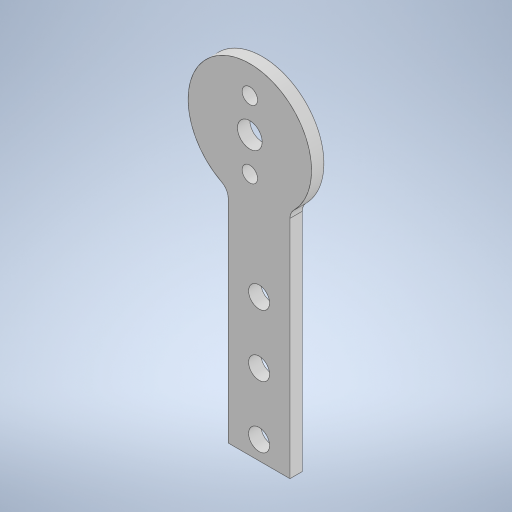
# Autodesk Inventor part: cutter_board_claws_endeffector_8_5_rotary-blade
Saved by Autodesk Inventor 2024 (Build 280153000, 153)
## iProperties
Created: 2025-06-01
Part Number: cutter_board_claws_endeffector_8_5_rotary-blade
Material: 一般
Document SubType Name: Modeling
Designer: 1412z
Density: 1 g/cm^3
Appearance: 既定
Author: 1412z
Autodesk Inventor part; units mm, degrees
ref_plane "YZ Plane" through (0, 0, 0) normal (1, 0, 0) x (0, 1, 0)
ref_plane "XZ Plane" through (0, 0, 0) normal (0, 1, 0) x (-1, 0, 0)
ref_plane "XY Plane" through (0, 0, 0) normal (0, 0, 1) x (1, 0, 0)
sketch "スケッチ1" plane through (0, 0, 0) normal (0, 0, 1) x (1, 0, 0)
  circle A0 centre (0, 0) radius 10
  line L0 (0, 0) -> (6.5, 0)
  line L1 (6.5, 0) -> (6.5, -45)
  line L2 (6.5, -45) -> (-3.5, -45)
  line L3 (-3.5, -45) -> (-3.5, 0)
  circle A1 centre (1.5, -22) radius 1.7
  circle A2 centre (1.5, -32) radius 1.7
  circle A3 centre (1.5, -42) radius 1.7
  circle A4 centre (0, 0) radius 5.5
  circle A5 centre (0, 5.5) radius 1.25
  circle A6 centre (0, -5.5) radius 1.25
  circle A7 centre (0, 0) radius 2
  point P0 (6.5, -7.5993)
  point P1 (-3.5, -9.3675)
  dimension "d0" = 20
  dimension "d3" = 6.5
  dimension "d4" = 45
  dimension "d5" = 10
  dimension "d6" = 3.4
  dimension "d7" = 3.4
  dimension "d8" = 3.4
  dimension "d9" = 11
  dimension "d10" = 2.5
  dimension "d11" = 2.5
  dimension "d12" = 4
  constraints: 8 centre point, 8 end point, 3 coincident, 3 perpendicular, 2 point on circle, 1 horizontal, 1 point on line
  measures "d0" diameter of A0
  measures "d3" distance of L0.start L0.end
  measures "d4" distance of L0.end L1.end
  measures "d5" distance of L1.end L2.end
  measures "d6" diameter of A1
  measures "d7" diameter of A2
  measures "d8" diameter of A3
  measures "d9" diameter of A4
  measures "d10" diameter of A5
  measures "d11" diameter of A6
  measures "d12" diameter of A7
extrude "押し出し1" add sketch "スケッチ1" along normal blind 2 contours A0 L1 L0 A4 A5 L3 | L3 A4 A6 L0 L1 A0 | A0 L1 L2 L3 | A4 A5 A6
fillet "フィレット1" radius 2 2 edges at (6.5, -7.5993, 1) (-3.5, -9.3675, 1)
